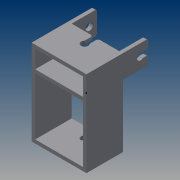
# Autodesk Inventor part: Box
Saved by Autodesk Inventor 2015 SP1 (Build 190203100, 203)
## iProperties
Created: 2015-04-28
Part Number: Box
Material: Generic
Document SubType Name: Modeling
Designer: Trevor
Density: 1 g/cm^3
Appearance: Default
Author: Trevor
Autodesk Inventor part; units mm, degrees
ref_plane "YZ Plane" through (0, 0, 0) normal (1, 0, 0) x (0, 1, 0)
ref_plane "XZ Plane" through (0, 0, 0) normal (0, 1, 0) x (-1, 0, 0)
ref_plane "XY Plane" through (0, 0, 0) normal (0, 0, 1) x (1, 0, 0)
sketch "Sketch1" plane through (0, 0, 0) normal (0, 0, 1) x (1, 0, 0)
  line L0 (-165.5097, 13.5202) -> (-165.5097, -5.7863) projected
  line L1 (-233.7722, -34.2331) -> (-233.7722, 3.8669) projected
  line L2 (-160.7472, 21.6107) -> (-233.7722, 21.6107)
  line L3 (-233.7722, 21.6107) -> (-233.7722, -92.4581)
  line L4 (-233.7722, -92.4581) -> (-160.7472, -92.4581)
  line L5 (-160.7472, -92.4581) -> (-160.7472, 21.6107)
  line L6 (-160.7472, -0.8956) -> (-160.7472, 8.6294) projected
  line L7 (-233.7722, -34.2331) -> (-233.7722, 3.8669) projected
  line L8 (-194.9086, -6.7331) -> (-197.4908, -6.7331) projected
  line L9 (-199.6108, 14.4669) -> (-197.0286, 14.4669) projected
  point P0 (0, 0)
  dimension "d1" = 7.1437
  dimension "d2" = 85.725
  constraints: 8 end point, 2 collinear, 2 parallel, 1 horizontal, 1 perpendicular
  measures "d1" distance between parallel lines of L2 L9
  measures "d2" distance between parallel lines of L4 L8
extrude "Extrusion1" add sketch "Sketch1" against normal blind 82.55
shell "Shell1" thickness 4.7625 removed faces 2 at (-185.0889, -54.4351, -82.55) at (-185.0889, -54.4351, 0)
sketch "Sketch2" plane through (0, 0, -82.55) normal (0, 0, -1) x (-1, 0, 0)
  line L0 (199.6108, -6.7331) -> (197.0286, -6.7331) projected
  line L1 (193.8921, -11.4956) -> (200.6273, -11.4956) projected
  line L2 (229.0097, 16.8482) -> (229.0097, -87.6956) projected
  line L3 (165.5097, -87.6956) -> (165.5097, 16.8482) projected
  line L4 (229.0097, -87.6956) -> (229.0097, 16.8482) projected
  line L5 (229.0097, -11.4956) -> (165.5097, -11.4956)
  line L6 (165.5097, -11.4956) -> (165.5097, -6.7331)
  line L7 (165.5097, -6.7331) -> (229.0097, -6.7331)
  line L8 (229.0097, -6.7331) -> (229.0097, -11.4956)
  point P0 (0, 0)
  constraints: 8 end point, 2 collinear, 2 parallel, 2 point on line, 1 horizontal, 1 perpendicular
extrude "Extrusion2" add sketch "Sketch2" against normal up to surface (82.55 mm away)
sketch "Sketch3" plane through (-233.7722, 21.6107, 0) normal (0, 1, 0) x (1, 0, 0)
  line L0 (73.025, 82.55) -> (0, 82.55) projected
  line L1 (36.5125, 82.55) -> (36.5125, 0)
  line L2 (0, 0) -> (73.025, 0) projected
  arc A0 (33.1449, 30.6087) -> (40.6772, 36.2864) centre (36.5125, 33.9763) ccw
  line L3 (73.025, 0) -> (0, 0) projected
  line L4 (33.1449, 30.6087) -> (39.8801, 30.6087)
  line L5 (39.8801, 30.6087) -> (39.8801, 37.3439)
  line L6 (39.8801, 37.3439) -> (33.1449, 37.3439)
  line L7 (33.1449, 37.3439) -> (33.1449, 30.6087)
  line L8 (33.1449, 30.6087) -> (39.8801, 37.3439) construction
  line L9 (39.8801, 30.6087) -> (33.1449, 37.3439) construction
  line L10 (39.8801, 37.3439) -> (39.8801, 39.3666)
  line L11 (33.1449, 37.3439) -> (33.1449, 39.3666)
  arc A1 (39.8801, 39.3666) -> (40.6772, 36.2864) centre (46.2301, 39.3666) ccw
  arc A2 (32.3478, 36.2864) -> (33.1449, 39.3666) centre (26.7949, 39.3666) ccw
  line L12 (68.2625, 82.55) -> (68.2625, 0) projected
  line L13 (4.7625, 0) -> (4.7625, 82.55) projected
  line L14 (4.7625, 82.55) -> (68.2625, 82.55)
  line L15 (68.2625, 82.55) -> (68.2625, 48.5832)
  line L16 (68.2625, 48.5832) -> (4.7625, 48.5832)
  line L17 (4.7625, 48.5832) -> (4.7625, 82.55)
  line L18 (33.1449, 39.3666) -> (33.1449, 82.55)
  arc A3 (32.3478, 36.2864) -> (33.1449, 30.6087) centre (36.5125, 33.9763) ccw
  line L19 (39.8801, 39.3666) -> (39.8801, 82.55)
  arc A4 (40.6772, 36.2864) -> (32.3478, 36.2864) centre (36.5125, 33.9763) ccw
  point P0 (233.7722, 0)
  dimension "d8" = 33.9763
  dimension "d9" = 6.7352
  dimension "d10" = 6.35
  dimension "d11" = 14.6069
  constraints: 30 end point, 14 point on circle, 7 perpendicular, 5 centre point, 4 midpoint, 4 parallel, 4 point on line, 3 symmetric about line, 3 tangent, 2 horizontal, 1 other
  measures "d8" distance from line of L3 A0.centre
  measures "d9" distance of L4.end L5.end
  measures "d10" radius of A1
  measures "d11" distance from line of A0.centre L16
extrude "Extrusion3" cut sketch "Sketch3" against normal through all contours L12 L16 L19 L0 | L19 L16 L1 L0 | L1 L16 L18 L0 | L19 L10 A4 L1 L16 | L18 L16 L13 L0 | L1 A4 L11 L18 L16 | A1 A4 L10 | A4 L6 L1 | L1 L6 A4 | A4 A0 L5 | L5 L4 L1 L6 | A0 L4 L1 | L1 L4 A0 | L11 A4 A2 | L1 L4 L7 L6 | L7 A3 A4
fillet "Fillet1" radius 3.175 6 edges at (-200.6273, 19.2294, -48.5832) (-193.8921, 19.2294, -48.5832) (-193.8921, -9.1143, -48.5832) (-200.6273, -9.1143, -48.5832) (-193.8921, -90.0768, -48.5832) (-200.6273, -90.0768, -48.5832)
sketch "Sketch4" plane through (-160.7472, -92.4581, 0) normal (1, 0, 0) x (0, 0, -1)
  point P0 (0, 92.4581)
sketch "Sketch5" plane through (-160.7472, -92.4581, 0) normal (1, 0, 0) x (0, 0, -1)
  circle A0 centre (72.0812, 98.7063) radius 4.7625 projected
  line L0 (68.7136, 95.3387) -> (75.4488, 95.3387) projected
  line L1 (75.4488, 102.0738) -> (68.7136, 102.0738) projected
  line L2 (75.4488, 95.3387) -> (82.55, 95.3387)
  line L3 (75.4488, 102.0738) -> (82.55, 102.0738)
  line L4 (76.8437, 98.7063) -> (67.3187, 98.7063)
  arc A1 (77.4716, 95.3387) -> (74.3914, 94.5416) centre (77.4716, 88.9887) ccw
  arc A2 (74.3914, 102.8709) -> (77.4716, 102.0738) centre (77.4716, 108.4238) ccw
  line L5 (82.55, 114.0688) -> (82.55, 0) projected
  point P0 (0, 92.4581)
  dimension "d15" = 6.35
  constraints: 6 end point, 4 point on circle, 3 horizontal, 3 point on line, 3 symmetric about line, 2 centre point, 1 midpoint, 1 tangent, 6 other
  measures "d15" radius of A1
extrude "Extrusion4" cut sketch "Sketch5" against normal through all contours L4 A0 L1 | A0 L0 L4 | L1 A0 | A0 L0
sketch "Sketch6" plane through (-160.7472, -92.4581, 0) normal (1, 0, 0) x (0, 0, -1)
  point P0 (0, 92.4581)
sketch "Sketch7" plane through (-160.7472, -92.4581, 0) normal (1, 0, 0) x (0, 0, -1)
  circle A0 centre (72.0812, 98.7063) radius 4.7625
  line L0 (68.7136, 95.3387) -> (75.4488, 95.3387)
  line L1 (75.4488, 102.0738) -> (68.7136, 102.0738)
  line L2 (75.4488, 95.3387) -> (82.55, 95.3387)
  line L3 (75.4488, 102.0738) -> (82.55, 102.0738)
  line L4 (76.8437, 98.7063) -> (67.3187, 98.7063)
  arc A1 (77.4716, 95.3387) -> (74.3914, 94.5416) centre (77.4716, 88.9887) ccw
  arc A2 (74.3914, 102.8709) -> (77.4716, 102.0738) centre (77.4716, 108.4238) ccw
  line L5 (68.7136, 95.3387) -> (75.4488, 95.3387) projected
  line L6 (75.4488, 102.0738) -> (68.7136, 102.0738) projected
  line L7 (82.55, 114.0688) -> (82.55, 0) projected
  point P0 (0, 92.4581)
  dimension "d18" = 6.35
  constraints: 6 end point, 4 point on circle, 3 horizontal, 3 point on line, 3 symmetric about line, 2 centre point, 1 midpoint, 1 tangent, 6 other
  measures "d18" radius of A1
extrude "Extrusion5" cut sketch "Sketch7" against normal up to next contours A0 L3 L7 L2
fillet "Fillet2" radius 3.175 2 edges at (-163.1285, 2.8806, -82.55) (-163.1285, 9.6158, -82.55)
sketch "Sketch8" plane through (-160.7472, -92.4581, 0) normal (1, 0, 0) x (0, 0, -1)
  arc A0 (62.5423, 86.8182) -> (84.9847, 90.5933) centre (72.0812, 98.7063) ccw projected
  line L0 (48.5832, 85.725) -> (48.5832, 80.9625) projected
  line L1 (0, 0) -> (82.55, 0) projected
  line L2 (82.55, 92.1637) -> (82.55, 0) projected
  line L3 (82.55, 83.4643) -> (48.5832, 83.4643)
  line L4 (48.5832, 83.4643) -> (48.5832, 0)
  line L5 (48.5832, 0) -> (82.55, 0)
  line L6 (82.55, 0) -> (82.55, 83.4643)
  point P0 (0, 92.4581)
  constraints: 8 end point, 2 parallel, 2 point on line, 1 collinear, 1 horizontal, 1 perpendicular, 1 tangent
extrude "Extrusion6" cut sketch "Sketch8" against normal through all contours L3 L2 L1 L4 L0
fillet "Fillet3" radius 3.175 4 edges at (-231.391, -8.9938, -82.55) (-231.391, 21.6107, -82.55) (-163.1285, 21.6107, -82.55) (-163.1285, -8.9938, -82.55)
equation "\"d1\" = 1.5 * t"
equation "\"d5\" = t"
equation "\"d8\" = r_gear + t"
equation "\"d9\" = l_key"
equation "\"d11\" = 0.5 * r_gear"
equation "\"t\" = 4.7625"
equation "\"r_gear\" = 29.213787"
equation "\"l_key\" = 6.735192"
body "Solid1"
